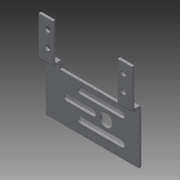
# Autodesk Inventor part: Side Servo Mount
Saved by Autodesk Inventor 2014 (Build 180170000, 170)
## iProperties
Created: 2013-11-16
Part Number: Side Servo Mount
Material: Generic
Document SubType Name: Modeling
Designer: Allison
Density: 1 g/cm^3
Appearance: Default
Author: Allison
Autodesk Inventor part; units mm, degrees
ref_plane "YZ Plane" through (0, 0, 0) normal (1, 0, 0) x (0, 1, 0)
ref_plane "XZ Plane" through (0, 0, 0) normal (0, 1, 0) x (-1, 0, 0)
ref_plane "XY Plane" through (0, 0, 0) normal (0, 0, 1) x (1, 0, 0)
sketch "Sketch1" plane through (0, 0, 0) normal (1, 0, 0) x (0, 1, 0)
  line L0 (0, 0) -> (32.73, 0)
  line L1 (34, 1.27) -> (34, 1.5875)
  line L2 (31.6505, 1.5875) -> (0, 1.5875)
  line L3 (0, 1.5875) -> (0, 0)
  line L4 (34, 6) -> (32.4125, 6)
  line L5 (32.4125, 4.73) -> (32.4125, 2.3495)
  line L6 (33.6825, 6) -> (57.8125, 6)
  line L7 (57.8125, 6) -> (57.8125, 4.4125)
  line L8 (57.8125, 4.4125) -> (34.762, 4.4125)
  arc A0 (34.762, 4.4125) -> (34, 3.6505) centre (34.762, 3.6505) ccw
  arc A1 (31.6505, 1.5875) -> (32.4125, 2.3495) centre (31.6505, 2.3495) ccw
  arc A2 (32.73, 0) -> (34, 1.27) centre (32.73, 1.27) ccw
  arc A3 (33.6825, 6) -> (32.4125, 4.73) centre (33.6825, 4.73) ccw
  line L9 (34, 3.6505) -> (34, 1.5875)
  point P0 (32.4125, 0)
  dimension "d0" = 34
  dimension "d1" = 1.5875
  dimension "d3" = 1.5875
  dimension "d4" = 25.4
  dimension "d5" = 1.5875
  dimension "d7" = 1.27
  constraints: 20 end point, 8 point on circle, 8 tangent, 5 perpendicular, 5 point on line, 4 centre point, 3 parallel, 1 equal radius, 1 horizontal
  measures "d0" distance of L2.end L1.end
  measures "d1" distance of L2.end L0.start
  measures "d3" distance of L4.start L4.end
  measures "d4" distance of L4.end L6.end
  measures "d5" distance of L6.end L7.end
  measures "d7" radius of A2
extrude "Extrusion1" add sketch "Sketch1" along normal blind 59
sketch "Sketch2" plane through (0, 57.8125, 6) normal (0, 1, 0) x (1, 0, 0)
  line L0 (0, 0) -> (59, 0) projected
  line L1 (0, 1.5875) -> (59, 1.5875) projected
  line L2 (0, 0) -> (9, 0)
  line L3 (59, 0) -> (50, 0)
  line L4 (50, 0) -> (9, 0)
  line L5 (9, 0) -> (9, 6.35)
  line L6 (9, 6.35) -> (50, 6.35)
  line L7 (50, 6.35) -> (50, 0)
  point P0 (0, 6)
  dimension "d10" = 9
  dimension "d11" = 9
  constraints: 12 end point, 2 parallel, 2 perpendicular, 2 point on line
  measures "d10" distance of L0.start L2.end
  measures "d11" distance of L0.end L3.end
extrude "Extrusion2" cut sketch "Sketch2" against normal blind 28.5
sketch "Sketch3" plane through (0, 0, 1.5875) normal (0, 0, 1) x (1, 0, 0)
  line L0 (50, 29.3125) -> (9, 29.3125) projected
  circle A0 centre (38.0547, 16) radius 4.0005
  line L1 (48.0547, 8) -> (22.0547, 8)
  line L2 (48.0547, 8) -> (22.0547, 8) construction
  line L3 (48.0547, 9.8542) -> (22.0547, 9.8542)
  line L4 (22.0547, 6.1458) -> (48.0547, 6.1458)
  arc A1 (48.0547, 6.1458) -> (48.0547, 9.8542) centre (48.0547, 8) ccw
  arc A2 (22.0547, 9.8542) -> (22.0547, 6.1458) centre (22.0547, 8) ccw
  line L5 (48.0547, 24) -> (22.0547, 24) construction
  line L6 (48.0547, 22.1458) -> (22.0547, 22.1458)
  line L7 (22.0547, 25.8542) -> (48.0547, 25.8542)
  arc A3 (48.0547, 22.1458) -> (48.0547, 25.8542) centre (48.0547, 24) ccw
  arc A4 (22.0547, 25.8542) -> (22.0547, 22.1458) centre (22.0547, 24) ccw
  line L8 (30.0547, 16) -> (13.0547, 16)
  line L9 (30.0547, 16) -> (13.0547, 16) construction
  line L10 (30.0547, 17.8669) -> (13.0547, 17.8669)
  line L11 (13.0547, 14.1331) -> (30.0547, 14.1331)
  arc A5 (30.0547, 14.1331) -> (30.0547, 17.8669) centre (30.0547, 16) ccw
  arc A6 (13.0547, 17.8669) -> (13.0547, 14.1331) centre (13.0547, 16) ccw
  point P0 (35.0547, 8)
  point P1 (21.5547, 16)
  dimension "d21" = 17
  dimension "d22" = 3.7338
  constraints: 28 end point, 12 point on circle, 8 tangent, 7 centre point, 4 parallel, 2 midpoint
  measures "d21" distance of L8.start L8.end
  measures "d22" diameter of A6
extrude "Extrusion3" cut sketch "Sketch3" against normal blind 28.5
sketch "Sketch4" plane through (0, 33.6825, 6) normal (0, 0, 1) x (1, 0, 0)
  line L0 (50, 24.13) -> (50, 0) projected
  line L1 (50, 0) -> (59, 0) projected
  line L2 (59, 24.13) -> (59, 0) projected
  line L3 (50, 24.13) -> (59, 24.13) projected
  circle A0 centre (5.4991, 18.13) radius 1.8542
  circle A1 centre (5.4991, 8.1224) radius 1.8542
  circle A2 centre (53.4991, 18.13) radius 1.8542
  circle A3 centre (53.4991, 8.1224) radius 1.8542
  point P0 (0, -33.6825)
  constraints: 4 centre point
extrude "Extrusion4" cut sketch "Sketch4" against normal blind 28.5 contours A0 | A1 | A2 | A3
body "Solid1"
